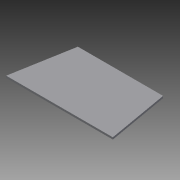
# Autodesk Inventor part: Panel_bottom
Saved by Autodesk Inventor 2013 (Build 170138000, 138)
## iProperties
Created: 2012-08-20
Part Number: Panel_bottom
Material: Generic
Document SubType Name: Modeling
Designer: Brandon
Density: 1 g/cm^3
Author: Brandon
Autodesk Inventor part; units mm, degrees
ref_plane "YZ Plane" through (0, 0, 0) normal (1, 0, 0) x (0, 1, 0)
ref_plane "XZ Plane" through (0, 0, 0) normal (0, 1, 0) x (-1, 0, 0)
ref_plane "XY Plane" through (0, 0, 0) normal (0, 0, 1) x (1, 0, 0)
sketch "Sketch1" plane through (0, 0, 0) normal (0, 1, 0) x (-1, 0, 0)
  line L0 (139.7346, -100) -> (-139.7346, -100)
  line L1 (-139.7346, -100) -> (-175, 100)
  line L2 (-175, 100) -> (175, 100)
  line L3 (175, 100) -> (139.7346, -100)
  point P0 (0, 0)
  point P1 (0, -100)
  point P2 (157.3673, 0)
  dimension "d0" = 80
  dimension "d1" = 80
  dimension "d2" = 350
  dimension "d4" = 200
  constraints: 8 end point, 2 midpoint, 1 horizontal, 1 horizontal alignment, 1 parallel, 1 vertical alignment
  measures "d0" angle of L2 L3
  measures "d1" angle of L2 L1
  measures "d2" distance of L1.end L2.end
  measures "d4" distance between parallel lines of L2 L0
extrude "Extrusion1" add sketch "Sketch1" along normal blind 6.35
body "Solid1"
